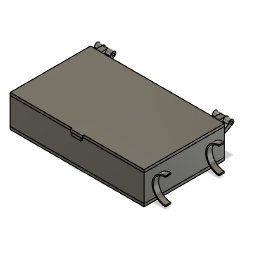
Component Box and Tool Kit v2 (Autodesk Fusion 360 design; units mm, degrees)
Autodesk Fusion 360 part; units mm, degrees
sketch "Sketch1" plane through (0, 0, 0) normal (0, 1, 0) x (1, 0, 0)
  line L0 (250, -150) -> (-250, -150)
  line L1 (-250, -150) -> (-250, 150)
  line L2 (-250, 150) -> (250, 150)
  line L3 (250, 150) -> (250, -150)
  line L4 (250, -150) -> (-250, 150) construction
  line L5 (-250, -150) -> (250, 150) construction
  dimension "d1" = 500
  dimension "d2" = 300
  constraint horizontal L0
  constraint perpendicular L0 L1
  constraint parallel L0 L2
  constraint parallel L1 L3
  constraint coincident L4 origin
  constraint coincident L5 origin
  measures "d1" distance of L0.start L0.end
  measures "d2" distance of L0.start L2.end
extrude "Extrude1" add sketch "Sketch1" along normal blind 10 makes body 1
sketch "Sketch2" plane through (0, 10, 0) normal (0, 1, 0) x (-1, 0, 0)
  line L0 (-250, -150) -> (250, -150)
  line L1 (250, -150) -> (250, 150)
  line L2 (250, 150) -> (-250, 150)
  line L3 (-250, 150) -> (-250, -150)
  line L4 (-250, 150) -> (250, 150)
  line L5 (250, 150) -> (250, -150)
  line L6 (250, -150) -> (-250, -150)
  line L7 (-250, -150) -> (-250, 150)
  line L8 (250, -150) -> (-250, -150)
  line L9 (-250, -150) -> (-250, 150)
  line L10 (-250, 150) -> (250, 150)
  line L11 (250, 150) -> (250, -150)
  line L12 (250, -150) -> (-250, 150) construction
  line L13 (-250, -150) -> (250, 150) construction
  line L14 (-245, -145) -> (-245, 145)
  line L15 (245, 145) -> (245, -145)
  line L16 (90, 145) -> (90, -145)
  line L17 (95, -145) -> (95, 145)
  line L18 (95, 145) -> (90, -145) construction
  line L19 (90, 145) -> (95, -145) construction
  line L20 (-245, 145) -> (90, 145)
  line L21 (95, 145) -> (245, 145)
  line L22 (245, -145) -> (95, -145)
  line L23 (90, -145) -> (-245, -145)
  point P0 (92.5, 0)
  dimension "d6" = 5
  dimension "d7" = 150
  constraint horizontal L4
  constraint vertical L5
  constraint horizontal L6
  constraint vertical L7
  constraint coincident L0.end L1.start
  constraint coincident L2.end L3.start
  constraint horizontal L8
  constraint perpendicular L8 L9
  constraint parallel L8 L10
  constraint parallel L9 L11
  constraint coincident L12 origin
  constraint coincident L13 origin
  constraint parallel L16 L17
  constraint coincident L18 P0
  constraint coincident L19 P0
  constraint parallel L8 L22
  constraint parallel L9 L14
  constraint parallel L10 L20
  constraint parallel L11 L15
  constraint collinear L20 L21
  constraint collinear L22 L23
  measures "d6" distance of L16.end L17.start
  measures "d7" distance of L15 L17
extrude "Extrude1'" add sketch "Sketch2" along normal blind 100 separate body makes body 2 in component "Component"
sketch "Sketch3" plane through (0, 110, 0) normal (0, 1, 0) x (-1, 0, 0)
  line L0 (245, 145) -> (245, -145)
  line L1 (245, -145) -> (95, -145)
  line L2 (95, -145) -> (95, 145)
  line L3 (95, 145) -> (245, 145)
  line L4 (90, 145) -> (90, -145)
  line L5 (90, -145) -> (-245, -145)
  line L6 (-245, -145) -> (-245, 145)
  line L7 (-245, 145) -> (90, 145)
  line L8 (250, 150) -> (-250, 150)
  line L9 (-250, 150) -> (-250, -150)
  line L10 (-250, -150) -> (250, -150)
  line L11 (250, -150) -> (250, 150)
  line L12 (-250, 150) -> (250, 150)
  line L13 (250, 150) -> (250, -150)
  line L14 (250, -150) -> (-250, -150)
  line L15 (-250, -150) -> (-250, 150)
  constraint horizontal L12
  constraint vertical L13
  constraint horizontal L14
  constraint vertical L15
  constraint coincident L10.end L11.start
  constraint coincident L8.end L9.start
extrude "Extrude2" add sketch "Sketch3" along normal blind 10 separate body contours L0 L1 L2 L3 | L4 L5 L6 L7 | L8 L9 L10 L11 L12 L13 L14 L15 makes body 3
sketch "Sketch4" plane through (250, 0, 0) normal (1, 0, 0) x (0, 0, -1)
  line L0 (-150, 10) -> (150, 10)
  line L1 (150, 10) -> (150, 110)
  line L2 (150, 110) -> (-150, 110)
  line L3 (-150, 110) -> (-150, 10)
  line L4 (175, 125) -> (175, 75) construction
  circle A0 centre (175, 110) radius 10
  circle A1 centre (175, 110) radius 5
  line L5 (150, 110) -> (175, 110) construction
  line L6 (179.5571, 101.0987) -> (150, 85.9665)
  line L7 (150, 120) -> (175, 120)
  line L8 (165.2081, 107.9704) -> (150, 101.1307)
  line L9 (165, 110) -> (150, 110)
  line L10 (150, 120) -> (150, 110)
  dimension "d12" = 25
  constraint vertical L4
  constraint coincident L4 A0.centre
  constraint concentric A0 A1
  constraint coincident L1.end L2.start
  constraint coincident A0.centre A1.centre
  constraint perpendicular L4 L5
  constraint coincident A0 L6.start
  constraint coincident L1 L6.end
  constraint tangent A0 L6
  constraint coincident A0 L7.end
  constraint tangent A0 L7
  constraint coincident A0 L8.start
  constraint coincident L1 L8.end
  constraint coincident A0 L9.start
  constraint coincident L5 L9.start
  constraint vertical L10
  measures "d12" distance of L1 L4
extrude "Extrude1''" add sketch "Sketch4" against normal blind 20 separate body contours L1 A0 L6 L8 | A0 makes body 4 in component "Component'"
extrude "Extrude3" add sketch "Sketch4" against normal blind 20 from surface at -20 contours A0 L7 L9 L10 | A0 bodies 3
extrude "Extrude4" add sketch "Sketch4" against normal blind 20 from surface at -40 contours L1 A0 L6 L8 | A0 bodies 3
extrude "Extrude2'" add sketch "Sketch4" along normal blind 20 from surface at -500 contours L1 A0 L6 L8 | A0 bodies 2 in component "Component"
extrude "Extrude5" add sketch "Sketch4" along normal blind 20 from surface at -480 contours A0 L7 L9 L10 | A0 bodies 3
extrude "Extrude6" add sketch "Sketch4" along normal blind 20 from surface at -460 contours L1 A0 L6 L8 | A0 bodies 3
sketch "Sketch5" plane through (0, 0, 150) normal (0, 0, 1) x (1, 0, 0)
  line L0 (-250, 110) -> (250, 110)
  line L1 (250, 110) -> (250, 120)
  line L2 (250, 120) -> (-250, 120)
  line L3 (-250, 120) -> (-250, 110)
  line L4 (-20, 120) -> (25, 120)
  line L5 (25, 120) -> (25, 100)
  line L6 (25, 100) -> (-20, 100)
  line L7 (-20, 100) -> (-20, 120)
  constraint horizontal L4
  constraint vertical L5
  constraint horizontal L6
  constraint vertical L7
  constraint coincident L2 L4.start
extrude "Extrude7" add sketch "Sketch5" along normal blind 5 contours L0 L2 L4 L5 L7 bodies 3
sketch "Sketch6" plane through (0, 0, 150) normal (0, 0, 1) x (1, 0, 0)
  line L0 (-250, 10) -> (250, 10)
  line L1 (250, 10) -> (250, 110)
  line L2 (250, 110) -> (-250, 110)
  line L3 (-250, 110) -> (-250, 10)
  line L4 (-15, 110) -> (20, 110)
  line L5 (20, 110) -> (20, 100)
  line L6 (20, 100) -> (-15, 100)
  line L7 (-15, 100) -> (-15, 110)
  constraint horizontal L4
  constraint vertical L5
  constraint horizontal L6
  constraint vertical L7
  constraint coincident L2 L4.start
extrude "Extrude1'''" add sketch "Sketch6" along normal blind 5 separate body contours L2 L4 L5 L6 L7 makes body 5 in component "Component''"
sketch "Sketch7" plane through (-250, 0, 0) normal (-1, 0, 0) x (0, 0, 1)
  circle A0 centre (-175, 110) radius 5
  line L0 (-150, 10) -> (150, 10)
  line L1 (150, 10) -> (150, 110)
  line L2 (150, 110) -> (-150, 110)
  line L3 (-150, 110) -> (-150, 101.1307)
  line L4 (-150, 101.1307) -> (-165.2081, 107.9704)
  arc A1 (-165.2081, 107.9704) -> (-179.5571, 101.0987) centre (-175, 110) ccw
  line L5 (-179.5571, 101.0987) -> (-150, 85.9665)
  line L6 (-150, 85.9665) -> (-150, 10)
hole "Hole1" at (-250, 19.908, -140.09) direction (1, 0, 0) diameter 10 depth 30 tip angle 118 bodies 2 in component "Component"
hole "Hole2" at (-250, 19.2401, -124.5518) direction (1, 0, 0) diameter 10 depth 40 tip angle 118 bodies 2 in component "Component"
sketch "Sketch8" plane through (0, 0, 150) normal (0, 0, 1) x (1, 0, 0)
  line L0 (-250, 10) -> (250, 10)
  line L1 (250, 10) -> (250, 110)
  line L2 (250, 110) -> (-250, 110)
  line L3 (-250, 110) -> (-250, 10)
  line L4 (250, 60) -> (350, 60) construction
  line L5 (300, 130) -> (300, 0) construction
  arc A0 (300, 110) -> (300, 10) centre (300, 60) ccw
  arc A1 (300, 105.5184) -> (300, 14.4816) centre (300, 60) ccw
  line L6 (300, 110) -> (300, 105.5184)
  line L7 (300, 14.4816) -> (300, 10)
  line L8 (300, 14.4816) -> (300, 10) construction
  constraint midpoint L1 L4.start
  constraint perpendicular L1 L4
  constraint midpoint L4 A0.centre
  constraint coincident L4.start A0
  constraint concentric A0 A1
  constraint vertical L5
  constraint coincident L5 A0.start
  constraint coincident L5 A1.start
  constraint coincident L5 A1.end
  constraint coincident L5 A0.end
extrude "Extrude8" add sketch "Sketch8" along normal blind 20 from surface at -50 separate body contours A0 A1 L6 L7 makes body 6
extrude "Extrude9" add sketch "Sketch8" along normal blind 20 from surface at -250 separate body contours A0 A1 L6 L7 makes body 7
component "Component" placed x (1, 0, 0) y (0, 1, 0) z (0, 0, 1) at (0, 0, 0)
component "Component'" placed x (1, 0, 0) y (0, 1, 0) z (0, 0, 1) at (0, 0, 0)
component "Component''" placed x (1, 0, 0) y (0, 1, 0) z (0, 0, 1) at (0, 0, 0)
